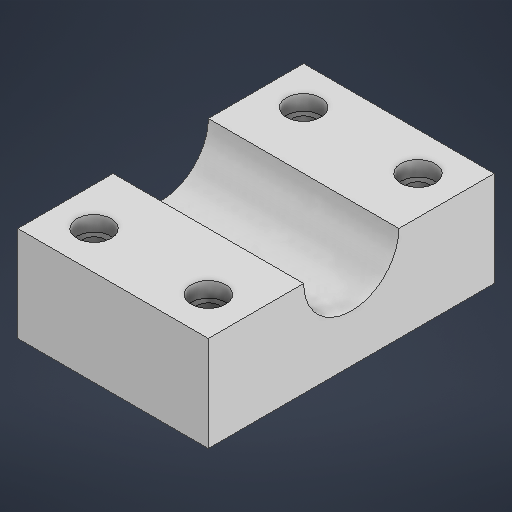
# Autodesk Inventor part: Part2
Saved by Autodesk Inventor 2026 (Build 300175050, 175E)
## iProperties
Created: 2026-04-16
Part Number: Part2
Material: Generic
Document SubType Name: Modeling
Designer: Administrator
Density: 1 g/cm^3
Appearance: Default
Author: Administrator
Autodesk Inventor part; units mm, degrees
ref_plane "YZ Plane" through (0, 0, 0) normal (1, 0, 0) x (0, 1, 0)
ref_plane "XZ Plane" through (0, 0, 0) normal (0, 1, 0) x (-1, 0, 0)
ref_plane "XY Plane" through (0, 0, 0) normal (0, 0, 1) x (1, 0, 0)
sketch "Sketch1" plane through (0, 0, 0) normal (1, 0, 0) x (0, 1, 0)
  line L0 (0, 0) -> (0, -150)
  line L1 (0, -150) -> (50, -150)
  line L2 (50, 0) -> (0, 0)
  arc A0 (50, -50) -> (50, -100) centre (50, -75) ccw
  line L3 (50, -150) -> (50, -100)
  line L4 (50, -50) -> (50, 0)
  dimension "d0" = 150
  dimension "d1" = 50
  dimension "d2" = 50
  constraints: 10 end point, 5 perpendicular, 2 point on circle, 1 centre point, 1 vertical
  measures "d0" distance of L0.start L0.end
  measures "d1" distance of L0.end L1.end
  measures "d2" diameter of A0
extrude "Extrusion1" add sketch "Sketch1" along normal mid plane 100
sketch "Sketch2" plane through (-50, 50, 0) normal (0, 1, 0) x (1, 0, 0)
  circle A0 centre (20, 20) radius 9
  circle A1 centre (20, 20) radius 6
  line L0 (0, 0) -> (0, 50) projected
  line L1 (100, 0) -> (0, 0) projected
  point P0 (50, 0)
  dimension "d5" = 18
  dimension "d6" = 12
  dimension "d7" = 20
  dimension "d8" = 20
  constraints: 2 centre point, 1 coincident
  measures "d5" diameter of A0
  measures "d6" diameter of A1
  measures "d7" distance from line of A0.centre L0
  measures "d8" distance from line of A0.centre L1
extrude "Extrusion2" cut sketch "Sketch2" against normal through all contours A1
extrude "Extrusion3" cut sketch "Sketch2" against normal blind 8
sketch "Sketch3" plane through (-50, 50, 0) normal (0, 1, 0) x (1, 0, 0)
  circle A0 centre (80, 20) radius 9
  circle A1 centre (80, 20) radius 6
  line L0 (100, 0) -> (0, 0) projected
  line L1 (100, 50) -> (100, 0) projected
  point P0 (50, 0)
  dimension "d13" = 18
  dimension "d14" = 12
  dimension "d15" = 20
  dimension "d16" = 20
  constraints: 2 centre point, 1 coincident
  measures "d13" diameter of A0
  measures "d14" diameter of A1
  measures "d15" distance from line of L0 A0.centre
  measures "d16" distance from line of L1 A0.centre
extrude "Extrusion4" cut sketch "Sketch3" against normal through all contours A1
extrude "Extrusion5" cut sketch "Sketch3" against normal blind 8
pattern_linear "Rectangular Pattern1" count 2 spacing 110 along (0, 0, -1) count 2 spacing -60 along (-1, 0, 0) of "Extrusion2", "Extrusion3"
body "Solid1"
